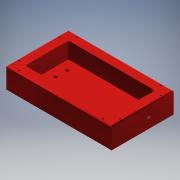
# Autodesk Inventor part: UNLHEP-14-01-P-004_ChuckForGantry
Saved by Autodesk Inventor 2019.4 (Build 234330000, 330)
## iProperties
Created: 2014-01-09
Part Number: UNLHEP-14-01-P-004_ChuckForGantry
Material: Aluminum, Anodized Red
Document SubType Name: Modeling
Designer: Frank Meier
Density: 2.7 g/cm^3
Project: UNL Pixel Phase I
Mass: 2699.72 g
Surface Area: 1115.91 cm^2
Volume: 999.896 cm^3
Appearance: Anodized - Red
Author: Frank Meier
Revision Number: 00
Autodesk Inventor part; units mm, degrees
ref_plane "YZ Plane" through (0, 0, 0) normal (1, 0, 0) x (0, 1, 0)
ref_plane "XZ Plane" through (0, 0, 0) normal (0, 1, 0) x (-1, 0, 0)
ref_plane "XY Plane" through (0, 0, 0) normal (0, 0, 1) x (1, 0, 0)
sketch "Skizze1" plane through (0, 0, 0) normal (0, 0, 1) x (1, 0, 0)
  line L0 (-117, -69) -> (117, -69)
  line L1 (117, -69) -> (117, 69)
  line L2 (117, 69) -> (-117, 69)
  line L3 (-117, 69) -> (-117, -69)
  line L4 (-117, -69) -> (117, 69) construction
  line L5 (117, -69) -> (-117, 69) construction
  point P0 (0, 0)
  dimension "d0" = 234
  dimension "d2" = 138
  constraints: 12 end point, 2 midpoint, 2 parallel, 1 horizontal, 1 perpendicular
  measures "d0" distance of L1.end L2.end
  measures "d2" distance of L0.end L1.end
extrude "Extrusion1" add sketch "Skizze1" along normal blind 46
sketch "Skizze2" plane through (0, 0, 46) normal (0, 0, 1) x (1, 0, 0)
  line L0 (-96, -48) -> (96, -48)
  line L1 (96, -48) -> (96, 48)
  line L2 (96, 48) -> (-96, 48)
  line L3 (-96, 48) -> (-96, -48)
  line L4 (-96, -48) -> (96, 48) construction
  line L5 (96, -48) -> (-96, 48) construction
  point P0 (0, 0)
  dimension "d5" = 192
  dimension "d7" = 96
  constraints: 12 end point, 2 midpoint, 2 parallel, 1 horizontal, 1 perpendicular
  measures "d5" distance of L1.end L2.end
  measures "d7" distance of L0.end L1.end
extrude "Extrusion2" cut sketch "Skizze2" against normal blind 36
fillet "Rundung1" radius 4 4 edges at (-96, 48, 28) (96, 48, 28) (96, -48, 28) (-96, -48, 28)
chamfer "Fase1" distance 2 angle 45 4 edges at (0, -69, 46) (-117, 0, 46) (0, 69, 46) (117, 0, 46)
sketch "Skizze4" plane through (0, 0, 46) normal (0, 0, 1) x (1, 0, 0)
  line L0 (117, 69) -> (-117, 69) projected
  line L1 (117, -69) -> (117, 69) projected
  line L2 (-117, 69) -> (-117, -69) projected
  line L3 (-117, -69) -> (117, -69) projected
  point P0 (-112, 45)
  point P1 (-112, -45)
  point P2 (-93, -64)
  point P3 (-93, 64)
  point P4 (93, 64)
  point P5 (112, 45)
  point P6 (112, -45)
  point P7 (93, -64)
  dimension "d153" = 24
  dimension "d154" = 24
  dimension "d155" = 5
  dimension "d156" = 5
  dimension "d157" = 24
  dimension "d158" = 5
  dimension "d159" = 5
  dimension "d160" = 24
  dimension "d161" = 24
  dimension "d162" = 5
  dimension "d163" = 5
  dimension "d164" = 24
  dimension "d165" = 5
  dimension "d166" = 24
  dimension "d167" = 5
  dimension "d168" = 24
  measures "d153" distance from line of L0 point (-112, 45)
  measures "d154" distance from line of L3 point (-112, -45)
  measures "d155" distance from line of L2 point (-112, -45)
  measures "d156" distance from line of L3 point (-93, -64)
  measures "d157" distance from line of L2 point (-93, -64)
  measures "d158" distance from line of L2 point (-112, 45)
  measures "d159" distance from line of L0 point (-93, 64)
  measures "d160" distance from line of L2 point (-93, 64)
  measures "d161" distance from line of L1 point (93, 64)
  measures "d162" distance from line of L0 point (93, 64)
  measures "d163" distance from line of L1 point (112, 45)
  measures "d164" distance from line of L0 point (112, 45)
  measures "d165" distance from line of L1 point (112, -45)
  measures "d166" distance from line of L3 point (112, -45)
  measures "d167" distance from line of L3 point (93, -64)
  measures "d168" distance from line of L1 point (93, -64)
hole "Bohrung7" at (-112, 45, 46) at (-112, -45, 46) at (-93, -64, 46) at (-93, 64, 46) at (93, 64, 46) at (112, 45, 46) at (112, -45, 46) at (93, -64, 46) direction (0, 0, -1) diameter 3.242 depth 20 tip angle 118 thread size "M4x0.7" class "6H" standard "ISO Metric profile"
sketch "Sketch12" plane through (0, 0, 10) normal (0, 0, 1) x (1, 0, 0)
  point P0 (0, 0)
  point P1 (76.2, 0)
  point P2 (-76.2, 0)
  point P3 (-76.2, 25.4)
  point P4 (76.2, 25.4)
  point P5 (76.2, -25.4)
  point P6 (-76.2, -25.4)
  dimension "d193" = 76.2
  dimension "d194" = 76.2
  dimension "d202" = 25.4
  dimension "d203" = 25.4
  dimension "d204" = 25.4
  dimension "d205" = 25.4
  constraints: 4 vertical alignment, 2 horizontal alignment
  measures "d193" distance of point (76.2, 0) point (0, 0)
  measures "d194" distance of point (0, 0) point (-76.2, 0)
  measures "d202" distance of point (-76.2, 25.4) point (-76.2, 0)
  measures "d203" distance of point (-76.2, 0) point (-76.2, -25.4)
  measures "d204" distance of point (76.2, 0) point (76.2, -25.4)
  measures "d205" distance of point (76.2, 0) point (76.2, 25.4)
hole "Hole9" at (76.2, 0, 10) at (-76.2, 0, 10) at (-76.2, 25.4, 10) at (-76.2, -25.4, 10) at (76.2, -25.4, 10) at (76.2, 25.4, 10) direction (0, 0, -1) diameter 6.756 end through all clearance for "Flat Head Machine Screw (82)" size "1/4" standard "Ansi Unified Screw Threads"
sketch "Sketch13" plane through (117, -69, 0) normal (1, 0, 0) x (0, 0, -1)
  line L0 (0, 138) -> (-44, 138) projected
  line L1 (0, 0) -> (0, 138) projected
  point P0 (0, 69)
  point P1 (-23, 83)
  dimension "d206" = 55
  dimension "d207" = 23
  measures "d206" distance from line of L0 point (-23, 83)
  measures "d207" distance from line of L1 point (-23, 83)
hole "Hole10" at (117, 14, 23) direction (-1, 0, 0) diameter 7.95 depth 21 tip angle 118 taper from width 8.7366 to width 8.304 over 6.924 thread size "1/8" designation "1/8 - 27 NPT" standard "NPT"
